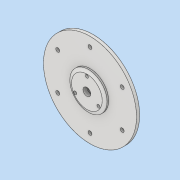
# Autodesk Inventor part: SpoolEndSpurSideLargeSpur
Saved by Autodesk Inventor 2017 (Build 210142000, 142)
## iProperties
Created: 2016-11-06
Part Number: SpoolEndSpurSideLargeSpur
Material: ABS Plastic
Document SubType Name: Modeling
Designer: techn
Density: 1.06 g/cm^3
Appearance: Smooth - White
Author: techn
Autodesk Inventor part; units mm, degrees
ref_plane "YZ Plane" through (0, 0, 0) normal (1, 0, 0) x (0, 1, 0)
ref_plane "XZ Plane" through (0, 0, 0) normal (0, 1, 0) x (-1, 0, 0)
ref_plane "XY Plane" through (0, 0, 0) normal (0, 0, 1) x (1, 0, 0)
sketch "Sketch1" plane through (0, 0, 0) normal (0, 0, 1) x (1, 0, 0)
  circle A0 centre (0, 0) radius 38.1
  dimension "d0" = 76.2
  constraints: 1 centre point, 1 coincident
  measures "d0" diameter of A0
extrude "Extrusion1" add sketch "Sketch1" along normal blind 2.54
sketch "Sketch5" plane through (0, 0, 2.54) normal (0, 0, 1) x (1, 0, 0)
  circle A0 centre (0, 0) radius 15.24
  dimension "d24" = 30.48
  constraints: 1 centre point, 1 coincident
  measures "d24" diameter of A0
extrude "Extrusion7" add sketch "Sketch5" along normal blind 2.54
sketch "Sketch6" plane through (0, 0, 5.08) normal (0, 0, 1) x (1, 0, 0)
  line L0 (0, 0) -> (0, 10.9985)
  circle A0 centre (0, 10.9985) radius 1.27
  circle A1 centre (-9.525, -5.4993) radius 1.27
  circle A2 centre (9.525, -5.4993) radius 1.27
  dimension "d28" = 2.54
  dimension "d31" = 360
  dimension "d49" = 19.05
  constraints: 3 centre point, 2 end point, 1 coincident, 1 vertical, 7 other
  measures "d28" diameter of A0
  measures "d49" distance of A2.centre L0.end
extrude "Extrusion8" cut sketch "Sketch6" against normal through all
sketch "Sketch7" plane through (0, 0, 5.08) normal (0, 0, 1) x (1, 0, 0)
  circle A0 centre (0, 0) radius 3.175
  dimension "d35" = 6.35
  constraints: 1 centre point, 1 coincident
  measures "d35" diameter of A0
extrude "Extrusion9" cut sketch "Sketch7" against normal blind 3.175
sketch "Sketch8" plane through (0, 0, 1.905) normal (0, 0, 1) x (1, 0, 0)
  circle A0 centre (0, 0) radius 2.3812
  dimension "d38" = 4.7625
  constraints: 1 centre point, 1 coincident
  measures "d38" diameter of A0
extrude "Extrusion10" cut sketch "Sketch8" against normal through all
sketch "Sketch9" plane through (0, 0, 2.54) normal (0, 0, 1) x (1, 0, 0)
  line L0 (0, 0) -> (0, 30.48)
  circle A0 centre (0, 30.48) radius 1.5875
  circle A1 centre (-26.3965, 15.24) radius 1.5875
  circle A2 centre (-26.3965, -15.24) radius 1.5875
  circle A3 centre (0, -30.48) radius 1.5875
  circle A4 centre (26.3965, -15.24) radius 1.5875
  circle A5 centre (26.3965, 15.24) radius 1.5875
  dimension "d41" = 30.48
  dimension "d42" = 3.175
  dimension "d45" = 360
  constraints: 6 centre point, 2 end point, 1 coincident, 1 vertical, 13 other
  measures "d41" distance of L0.start L0.end
  measures "d42" diameter of A0
extrude "Extrusion11" cut sketch "Sketch9" against normal blind 25.4
chamfer "Chamfer1" distance 2.667 distance2 1.27 1 edges at (-15.24, 0, 5.08) measured on face at (4.9695, 7.5399, 5.08)
body "Solid1"
